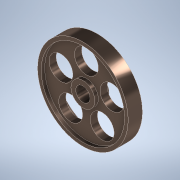
# Autodesk Inventor part: 8. 車輪
Saved by Autodesk Inventor 2022 (Build 260153000, 153)
## iProperties
Created: 2023-05-26
Part Number: 8. 車輪
Material: 一般
Document SubType Name: Modeling
Designer: USER
Density: 1 g/cm^3
Appearance: 砲銅 - 古董色拋光
Author: USER
Autodesk Inventor part; units mm, degrees
ref_plane "YZ Plane" through (0, 0, 0) normal (1, 0, 0) x (0, 1, 0)
ref_plane "XZ Plane" through (0, 0, 0) normal (0, 1, 0) x (-1, 0, 0)
ref_plane "XY Plane" through (0, 0, 0) normal (0, 0, 1) x (1, 0, 0)
sketch "草圖1" plane through (0, 0, 0) normal (1, 0, 0) x (0, 1, 0)
  line L0 (0, 0) -> (0, 54.3739) construction
  line L1 (0, 0) -> (54.3739, 0) construction
  line L2 (6, 6) -> (6, -6)
  line L3 (38, -6) -> (38, 6)
  line L4 (35, 3) -> (10, 3)
  line L5 (10, 6) -> (10, -6)
  line L6 (10, -3) -> (35, -3)
  line L7 (35, -6) -> (35, 6)
  line L8 (38, 6) -> (35, 6)
  line L9 (10, 6) -> (6, 6)
  line L10 (6, -6) -> (10, -6)
  line L11 (35, -6) -> (38, -6)
  dimension "d2" = 12
  dimension "d3" = 3
  dimension "d4" = 6
  dimension "d5" = 10
  dimension "d6" = 35
  dimension "d7" = 38
  dimension "d8" = 12
  constraints: 24 end point, 7 parallel, 4 horizontal, 4 point on line, 3 perpendicular, 1 vertical, 3 other
  measures "d2" distance between parallel lines of L11 L8
  measures "d3" distance between parallel lines of L4 L8
  measures "d4" distance between parallel lines of L2 L0
  measures "d5" distance between parallel lines of L5 L0
  measures "d6" distance between parallel lines of L7 L0
  measures "d7" distance between parallel lines of L0 L3
  measures "d8" distance between parallel lines of L10 L9
revolve "迴轉1" add sketch "草圖1" angle 360 about axis through (0, 0, 0) along (0, 0, 1)
sketch "草圖2" plane through (0, 0, 3) normal (0, 0, 1) x (1, 0, 0)
  circle A0 centre (0, 22.5) radius 10
  point P0 (0, 0)
  dimension "d10" = 20
  dimension "d11" = 22.5
  constraints: 1 centre point
  measures "d10" diameter of A0
  measures "d11" distance of point (0, 0) A0.centre
extrude "擠出1" cut sketch "草圖2" against normal through all
pattern_circular "環形陣列1" count 5 over 360 about axis through (0, 0, -10) along (0, 0, 1) of "擠出1"
